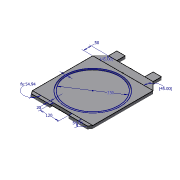
# Autodesk Inventor part: Base
Saved by Autodesk Inventor 2015 (Build 190159000, 159)
## iProperties
Created: 2020-04-22
Part Number: Base
Material: Generic
Document SubType Name: Modeling
Designer: Ghassan Yusuf
Density: 1 g/cm^3
Appearance: Default
Author: Ghassan Yusuf
Autodesk Inventor part; units mm, degrees
ref_plane "YZ Plane" through (0, 0, 0) normal (1, 0, 0) x (0, 1, 0)
ref_plane "XZ Plane" through (0, 0, 0) normal (0, 1, 0) x (-1, 0, 0)
ref_plane "XY Plane" through (0, 0, 0) normal (0, 0, 1) x (1, 0, 0)
sketch "Sketch1" plane through (0, 0, 0) normal (0, 0, 1) x (1, 0, 0)
  circle A0 centre (0, 0) radius 165
  circle A1 centre (0, 0) radius 175
  line L0 (-192.9296, 192.9296) -> (192.9296, 192.9296)
  line L1 (192.9296, 192.9296) -> (192.9296, -192.9296)
  line L2 (192.9296, -192.9296) -> (-192.9296, -192.9296)
  line L3 (-192.9296, -192.9296) -> (-192.9296, 192.9296)
  line L4 (-192.9296, -192.9296) -> (-178.8933, -212.9296)
  line L5 (-178.8933, -212.9296) -> (178.8933, -212.9296)
  line L6 (178.8933, -212.9296) -> (192.9296, -192.9296)
  line L7 (-192.9296, 192.9296) -> (-142.9296, 242.9296)
  line L8 (-142.9296, 242.9296) -> (142.9296, 242.9296)
  line L9 (142.9296, 242.9296) -> (192.9296, 192.9296)
  line L10 (-142.9296, 242.9296) -> (-92.9296, 242.9296)
  line L11 (-92.9296, 242.9296) -> (-92.9296, 292.9296)
  line L12 (-92.9296, 292.9296) -> (-142.9296, 292.9296)
  line L13 (-142.9296, 292.9296) -> (-142.9296, 242.9296)
  line L14 (142.9296, 242.9296) -> (92.9296, 242.9296)
  line L15 (92.9296, 242.9296) -> (92.9296, 292.9296)
  line L16 (92.9296, 292.9296) -> (142.9296, 292.9296)
  line L17 (142.9296, 292.9296) -> (142.9296, 242.9296)
  line L18 (-60, -212.9296) -> (60, -212.9296)
  line L19 (60, -212.9296) -> (60, -192.9296)
  line L20 (60, -192.9296) -> (-60, -192.9296)
  line L21 (-60, -192.9296) -> (-60, -212.9296)
  circle A2 centre (0, 0) radius 185
  circle A3 centre (0, 0) radius 180
  circle A4 centre (0, 0) radius 188
  point P0 (0, 192.9296)
  point P1 (-192.9296, 0)
  point P2 (0, 242.9296)
  point P3 (0, -212.9296)
  dimension "d0" = 330
  dimension "d1" = 10
  dimension "d2" = 54.938
  dimension "d3" = 54.938
  dimension "d4" = 20
  dimension "d5" = 45
  dimension "d6" = 45
  dimension "d7" = 50
  dimension "d12" = 120
  dimension "d15" = 10
  dimension "d16" = 5
  dimension "d21" = 3
  dimension "d27" = 50
  constraints: 44 end point, 9 parallel, 5 centre point, 5 horizontal, 5 perpendicular, 4 equal length, 4 midpoint, 3 point on line, 3 vertical alignment, 1 coincident, 1 horizontal alignment
  measures "d0" diameter of A0
  measures "d1" radial gap between concentric circles of A0 A1
  measures "d2" angle of L2 L6
  measures "d3" angle of L2 L4
  measures "d4" distance between parallel lines of L5 L2
  measures "d5" angle of L0 L7
  measures "d6" angle of L9 L0
  measures "d7" distance between parallel lines of L0 L8
  measures "d12" distance between parallel lines of L19 L21
  measures "d15" radial gap between concentric circles of A1 A2
  measures "d16" radial gap between concentric circles of A1 A3
  measures "d21" radial gap between concentric circles of A2 A4
  measures "d27" distance between parallel lines of L11 L13
extrude "Extrusion1" add sketch "Sketch1" against normal blind 18 contours A0 | A1 | L7 L8 L9 L0 | L0 L1 L2 L3 | L2 L21 L5 L4 | L13 L12 L11 L8 | L6 L5 L19 L2 | L8 L15 L16 L17 | L2 L19 L5 L21 | A2 | A3 | A4
extrude "Extrusion2" cut sketch "Sketch1" against normal blind 12 contours A0 | A1
extrude "Extrusion3" cut sketch "Sketch1" against normal blind 18 contours L2 L19 L5 L21
extrude "Extrusion4" cut sketch "Sketch1" against normal blind 15 contours A2
extrude "Extrusion5" cut sketch "Sketch1" against normal blind 10 contours A3
extrude "Extrusion6" cut sketch "Sketch1" against normal blind 2 contours A4
chamfer "Chamfer1" distance 20 angle 45 2 edges at (-60, -212.9296, -9) (60, -212.9296, -9)
equation "\"d3\" = d2"
body "Solid1"
